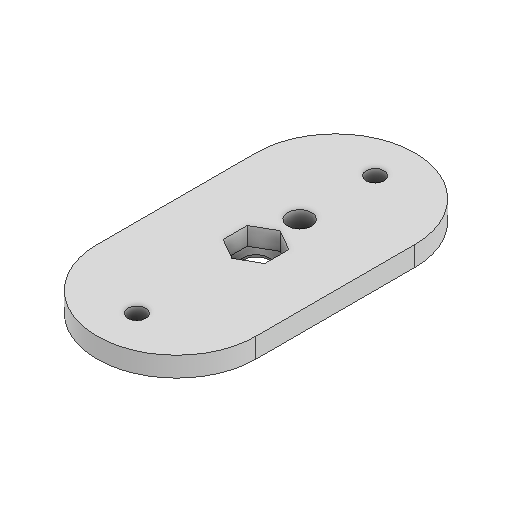
# Autodesk Inventor part: Tripod mount
Saved by Autodesk Inventor 2025.2 (Build 292293000, 293)
## iProperties
Created: 2025-07-08
Part Number: Tripod mount
Material: Generic
Document SubType Name: Modeling
Designer: rolan
Density: 1 g/cm^3
Appearance: Default
Author: rolan
Autodesk Inventor part; units mm, degrees
ref_plane "YZ Plane" through (0, 0, 0) normal (1, 0, 0) x (0, 1, 0)
ref_plane "XZ Plane" through (0, 0, 0) normal (0, 1, 0) x (-1, 0, 0)
ref_plane "XY Plane" through (0, 0, 0) normal (0, 0, 1) x (1, 0, 0)
sketch "Sketch1" plane through (0, 0, 0) normal (0, 1, 0) x (-1, 0, 0)
  line L0 (0, 40) -> (0, 40)
  line L1 (-20, 20) -> (-20, -20)
  line L2 (0, -40) -> (0, -40)
  line L3 (20, -20) -> (20, 20)
  line L4 (20, 40) -> (-20, -40) construction
  line L5 (-20, 40) -> (20, -40) construction
  arc A0 (0, -40) -> (20, -20) centre (0, -20) ccw
  arc A1 (20, 20) -> (0, 40) centre (0, 20) ccw
  arc A2 (0, 40) -> (-20, 20) centre (0, 20) ccw
  arc A3 (-20, -20) -> (0, -40) centre (0, -20) ccw
  point P0 (0, 0)
  dimension "d0" = 40
  dimension "d1" = 80
  dimension "d18" = 20
  constraints: 12 end point, 8 point on circle, 8 point on line, 8 tangent, 4 centre point, 2 equal radius, 2 midpoint, 2 parallel, 1 concentric, 1 horizontal, 1 perpendicular
  measures "d0" distance of L5.end L4.end
  measures "d1" distance of L4.end L5.start
  measures "d18" radius of A0
extrude "Extrusion1" add sketch "Sketch1" along normal blind 5
sketch "Sketch2" plane through (0, 5, 0) normal (0, 1, 0) x (1, 0, 0)
  line L0 (-5.25, 3.0311) -> (0, 6.0622)
  line L1 (0, 6.0622) -> (5.25, 3.0311)
  line L2 (5.25, 3.0311) -> (5.25, -3.0311)
  line L3 (5.25, -3.0311) -> (0, -6.0622)
  line L4 (0, -6.0622) -> (-5.25, -3.0311)
  line L5 (-5.25, -3.0311) -> (-5.25, 3.0311)
  point P0 (0, 0)
  point P1 (0, 0)
  point P2 (5.25, 0)
  point P3 (-5.25, 0)
  dimension "d4" = 10.5
  constraints: 12 end point, 2 midpoint, 1 coincident, 13 other
  measures "d4" distance of point (5.25, 0) point (-5.25, 0)
extrude "Extrusion2" cut sketch "Sketch2" against normal blind 4.5
sketch "Sketch3" plane through (0, 0.5, 0) normal (0, 1, 0) x (1, 0, 0)
  circle A0 centre (0, 0) radius 3.25
  dimension "d7" = 6.5
  constraints: 1 centre point, 1 coincident
  measures "d7" diameter of A0
extrude "Extrusion3" cut sketch "Sketch3" against normal through all
sketch "Sketch4" plane through (0, 0, 0) normal (0, -1, 0) x (1, 0, 0)
  circle A0 centre (0, -11) radius 3
  circle A1 centre (0, 30) radius 2.25
  circle A2 centre (0, -30) radius 2.25
  point P0 (0, 0)
  dimension "d10" = 6
  dimension "d11" = 11
  dimension "d12" = 4.5
  dimension "d13" = 4.5
  dimension "d14" = 30
  dimension "d15" = 30
  constraints: 3 centre point
  measures "d10" diameter of A0
  measures "d11" distance of A0.centre point (0, 0)
  measures "d12" diameter of A1
  measures "d13" diameter of A2
  measures "d14" distance of A1.centre point (0, 0)
  measures "d15" distance of A2.centre point (0, 0)
extrude "Extrusion4" cut sketch "Sketch4" against normal through all
body "Solid1"
